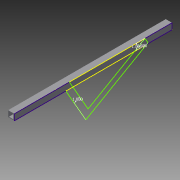
# Autodesk Inventor part: bar
Saved by Autodesk Inventor 2013 (Build 170138000, 138)
## iProperties
Created: 2013-03-02
Part Number: bar
Material: Generic
Document SubType Name: Modeling
Designer: Arpan
Density: 1 g/cm^3
Author: Arpan
Autodesk Inventor part; units mm, degrees
ref_plane "YZ Plane" through (0, 0, 0) normal (1, 0, 0) x (0, 1, 0)
ref_plane "XZ Plane" through (0, 0, 0) normal (0, 1, 0) x (-1, 0, 0)
ref_plane "XY Plane" through (0, 0, 0) normal (0, 0, 1) x (1, 0, 0)
sketch "Sketch1" plane through (0, 0, 0) normal (0, 0, 1) x (1, 0, 0)
  line L0 (0, 0) -> (-25.4, 0)
  line L1 (-25.4, 0) -> (-25.4, 25.4)
  line L2 (-25.4, 25.4) -> (0, 25.4)
  line L3 (0, 25.4) -> (0, 0)
  line L4 (-3.175, 22.225) -> (-22.225, 22.225)
  line L5 (-22.225, 22.225) -> (-22.225, 3.175)
  line L6 (-22.225, 3.175) -> (-3.175, 3.175)
  line L7 (-3.175, 3.175) -> (-3.175, 22.225)
  dimension "d0" = 25.4
  dimension "d2" = 25.4
  dimension "d3" = 3.175
  constraints: 16 end point, 4 parallel, 2 perpendicular, 1 horizontal, 3 other
  measures "d0" distance of L0.end L1.end
  measures "d2" distance of L1.end L2.end
  measures "d3" distance between parallel lines of L2 L4
extrude "Extrusion1" add sketch "Sketch1" along normal blind 660.4
sketch "Sketch2" plane through (0, 0, 0) normal (1, 0, 0) x (0, 0, -1)
  line L0 (0, 25.4) -> (0, 0) projected
  line L1 (0, 25.4) -> (-660.4, 25.4) projected
  line L2 (-660.4, 0) -> (-660.4, 25.4) projected
  line L3 (0, 0) -> (-660.4, 0) projected
  line L4 (-113.1604, 25.4) -> (-351.652, -111.264)
  line L5 (-351.652, -111.264) -> (-415.4102, 0)
  line L6 (-113.1604, 0) -> (0, 0)
  line L7 (-113.1604, 25.4) -> (0, 25.4)
  line L8 (0, 25.4) -> (0, 0)
  line L9 (-444.6849, 0) -> (-660.4, 0)
  line L10 (-660.4, 0) -> (-660.4, 25.4)
  line L11 (-660.4, 25.4) -> (-429.9653, 25.4)
  line L12 (-429.9653, 25.4) -> (-415.4102, 0)
  line L13 (-113.1604, 25.4) -> (-100.5318, 3.3619)
  line L14 (-100.5318, 3.3619) -> (-361.0615, -145.9308)
  line L15 (-361.0615, -145.9308) -> (-444.6849, 0)
  dimension "d6" = 25.4
  dimension "d9" = 25.4
  dimension "d12" = 25.4
  constraints: 24 end point, 5 point on line, 4 collinear, 3 perpendicular, 1 parallel
  measures "d6" distance of L4.start L6.start
  measures "d9" distance of L4.start L13.end
  measures "d12" distance between parallel lines of L5 L15
body "Solid1"
